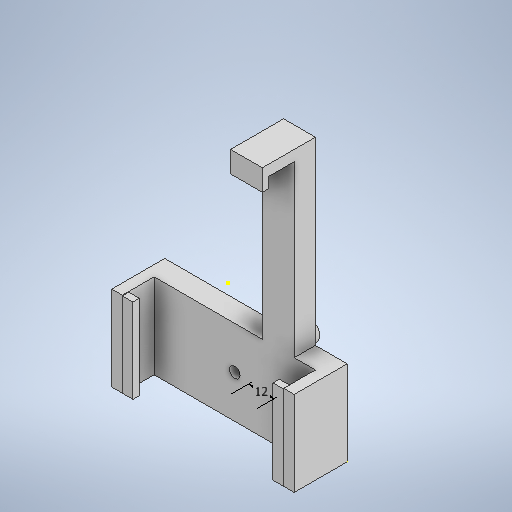
# Autodesk Inventor part: Holder
Saved by Autodesk Inventor 2025 (Build 290162000, 162)
## iProperties
Created: 2025-10-12
Part Number: Holder
Material: Generic
Document SubType Name: Modeling
Designer: parsh
Density: 1 g/cm^3
Appearance: Default
Author: parsh
Autodesk Inventor part; units mm, degrees
ref_plane "YZ Plane" through (0, 0, 0) normal (1, 0, 0) x (0, 1, 0)
ref_plane "XZ Plane" through (0, 0, 0) normal (0, 1, 0) x (-1, 0, 0)
ref_plane "XY Plane" through (0, 0, 0) normal (0, 0, 1) x (1, 0, 0)
sketch "Sketch1" plane through (0, 0, 0) normal (0, 0, 1) x (1, 0, 0)
  circle A0 centre (0, 0) radius 5
  circle A1 centre (0, 0) radius 2.5
  dimension "d0" = 10
  dimension "d1" = 5
  constraints: 2 centre point, 2 coincident
  measures "d0" diameter of A0
  measures "d1" diameter of A1
extrude "Extrusion1" add sketch "Sketch1" along normal blind 25
sketch "Sketch2" plane through (0, 0, 25) normal (0, 0, 1) x (1, 0, 0)
  line L0 (0, 20) -> (38, 20)
  line L1 (38, 20) -> (38, -20)
  line L2 (38, -20) -> (-38, -20)
  line L3 (-38, -20) -> (-38, 20)
  line L4 (-38, 20) -> (0, 20)
  circle A0 centre (0, 0) radius 2.5
  dimension "d4" = 20
  dimension "d6" = 38
  dimension "d7" = 40
  dimension "d8" = 76
  dimension "d9" = 40
  constraints: 10 end point, 2 perpendicular, 1 centre point, 1 coincident, 1 collinear, 1 horizontal, 1 point on line
  measures "d4" distance of point (0, 0) L0.start
  measures "d6" distance of L0.start L0.end
  measures "d7" distance of L0.end L1.end
  measures "d8" distance of L1.end L2.end
  measures "d9" distance of L2.end L3.end
extrude "Extrusion2" add sketch "Sketch2" along normal blind 10
sketch "Sketch3" plane through (0, 0, 35) normal (0, 0, 1) x (1, 0, 0)
  line L0 (38, 20) -> (-38, 20) projected
  line L1 (38, 20) -> (43, 20)
  line L2 (43, 20) -> (43, -20)
  line L3 (43, -20) -> (38, -20)
  line L4 (38, -20) -> (38, 20)
  line L5 (-38, 20) -> (-38, -20) projected
  line L6 (-38, -20) -> (-43, -20)
  line L7 (-43, -20) -> (-43, 20)
  line L8 (-43, 20) -> (-38, 20)
  line L9 (-38, 20) -> (-38, -20)
  point P0 (0, 0)
  dimension "d12" = 5
  dimension "d13" = 40
  dimension "d14" = 5
  constraints: 16 end point, 4 parallel, 2 horizontal, 2 perpendicular
  measures "d12" distance of L2.end L3.end
  measures "d13" distance of L1.end L2.end
  measures "d14" distance of L7.end L8.end
extrude "Extrusion3" add sketch "Sketch3" along normal blind 15 and the other way blind 10
sketch "Sketch4" plane through (-38, -20, 35) normal (1, 0, 0) x (0, 0, -1)
  point P0 (35, 20)
sketch "Sketch5" plane through (-38, -20, 35) normal (1, 0, 0) x (0, 0, -1)
  line L0 (0, 0) -> (-15, 0) projected
  line L1 (-14.9948, 39.7098) -> (-11.9948, 39.7098)
  line L2 (-11.9948, 39.7098) -> (-11.9948, 0)
  line L3 (-11.9948, 0) -> (-14.9948, 0)
  line L4 (-14.9948, 0) -> (-14.9948, 39.7098)
  point P0 (35, 20)
  dimension "d19" = 3
  constraints: 8 end point, 2 parallel, 1 horizontal, 1 perpendicular, 1 point on line
  measures "d19" distance of L2.end L3.end
extrude "Extrusion4" add sketch "Sketch5" along normal blind 5
sketch "Sketch6" plane through (38, -20, 35) normal (-1, 0, 0) x (0, 0, 1)
  line L0 (11.9948, 39.7098) -> (14.9948, 39.7098) projected
  line L1 (11.9948, 39.7098) -> (11.9948, 0) projected
  line L2 (14.9948, 39.7098) -> (11.9948, 39.7098)
  line L3 (11.9948, 39.7098) -> (11.9948, 0)
  line L4 (11.9948, 0) -> (14.9948, 0)
  line L5 (14.9948, 0) -> (14.9948, 39.7098)
  point P0 (-35, 20)
  constraints: 8 end point, 2 parallel, 1 horizontal, 1 perpendicular
extrude "Extrusion5" add sketch "Sketch6" along normal blind 5
sketch "Sketch11" plane through (-43, 20, 25) normal (0, 1, 0) x (1, 0, 0)
  line L0 (5, -10) -> (81, -10) projected
  line L1 (86, 0) -> (0, 0) projected
  line L2 (56, -10) -> (71, -10)
  line L3 (71, -10) -> (71, 0)
  line L4 (71, 0) -> (56, 0)
  line L5 (56, 0) -> (56, -10)
  point P0 (43, 25)
  dimension "d39" = 15
  constraints: 8 end point, 2 parallel, 2 point on line, 1 horizontal, 1 perpendicular
  measures "d39" distance of L4.end L3.end
extrude "Extrusion8" add sketch "Sketch11" along normal blind 85
sketch "Sketch12" plane through (0, 0, 35) normal (0, 0, 1) x (1, 0, 0)
  line L0 (13, 20) -> (13, 105) projected
  line L1 (13, 105) -> (13, 100)
  line L2 (13, 100) -> (28, 100)
  line L3 (28, 100) -> (28, 105)
  line L4 (28, 105) -> (13, 105)
  point P0 (0, 0)
  dimension "d42" = 5
  dimension "d43" = 15
  constraints: 8 end point, 3 perpendicular, 1 point on line
  measures "d42" distance of L0.end L1.end
  measures "d43" distance of L1.end L2.end
extrude "Extrusion9" add sketch "Sketch12" along normal blind 15
sketch "Sketch13" plane through (13, 100, 35) normal (0, -1, 0) x (1, 0, 0)
  line L0 (0, -10) -> (0, 15) projected
  line L1 (0, 15) -> (0, 12)
  line L2 (0, 12) -> (15, 12)
  line L3 (15, 12) -> (15, 15)
  line L4 (15, 15) -> (0, 15)
  point P0 (-13, -35)
  dimension "d46" = 3
  dimension "d47" = 15
  constraints: 8 end point, 3 perpendicular, 1 point on line
  measures "d46" distance of L0.end L1.end
  measures "d47" distance of L1.end L2.end
extrude "Extrusion10" add sketch "Sketch13" along normal blind 5
sketch "Sketch14" plane through (-43, -20, 25) normal (0, -1, 0) x (1, 0, 0)
  line L0 (0, 0) -> (86, 0) projected
  line L1 (43, 0) -> (31, 0)
  point P0 (43, -25)
  point P1 (56, 0)
  dimension "d50" = 12
  constraints: 2 end point, 1 midpoint, 1 point on line
  measures "d50" distance of L1.start L1.end
sketch "Sketch15" plane through (-43, -20, 25) normal (0, -1, 0) x (1, 0, 0)
  line L0 (48, 0) -> (38, 0) projected
  line L1 (43, 0) -> (31, 0)
  line L2 (31, 0) -> (31, 3)
  line L3 (31, 3) -> (16, 3)
  line L4 (16, 3) -> (16, 7)
  line L5 (16, 7) -> (31, 7)
  line L6 (31, 7) -> (31, 3)
  point P0 (43, -25)
  dimension "d51" = 12
  dimension "d52" = 3
  dimension "d53" = 15
  dimension "d54" = 4
  constraints: 12 end point, 2 parallel, 2 perpendicular, 1 collinear, 1 horizontal, 1 midpoint
  measures "d51" distance of L1.start L1.end
  measures "d52" distance of L1.end L2.end
  measures "d53" distance of L4.end L5.end
  measures "d54" distance of L3.end L4.end
extrude "Extrusion11" cut sketch "Sketch15" against normal blind 15
body "Solid1"
